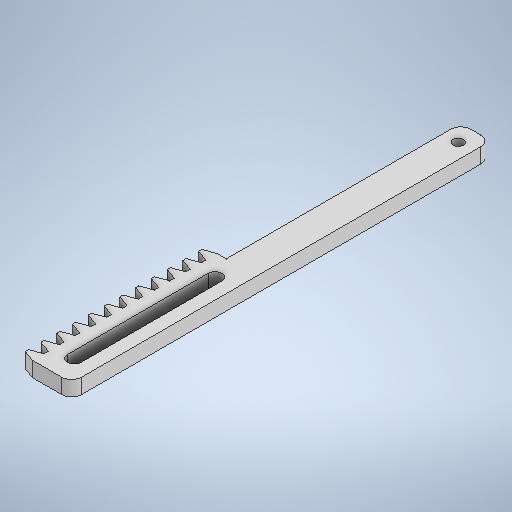
# Autodesk Inventor part: cremallera_v2
Saved by Autodesk Inventor 2025.2 (Build 292293000, 293)
## iProperties
Created: 2025-04-03
Part Number: cremallera_v2
Material: Generic
Document SubType Name: Modeling
Designer: cdavi
Density: 1 g/cm^3
Appearance: Default
Author: cdavi
Autodesk Inventor part; units mm, degrees
ref_plane "YZ Plane" through (0, 0, 0) normal (1, 0, 0) x (0, 1, 0)
ref_plane "XZ Plane" through (0, 0, 0) normal (0, 1, 0) x (-1, 0, 0)
ref_plane "XY Plane" through (0, 0, 0) normal (0, 0, 1) x (1, 0, 0)
sketch "Sketch1" plane through (0, 0, 0) normal (0, 1, 0) x (-1, 0, 0)
  line L0 (4.808, 48.5926) -> (7.058, 47.7737)
  line L1 (4.808, 49.4815) -> (4.808, 48.5926)
  line L2 (4.808, 49.4815) -> (7.058, 50.2996)
  line L3 (7.058, 50.2996) -> (7.058, 50.9144)
  line L4 (4.808, 51.7333) -> (7.058, 50.9144)
  line L5 (4.808, 52.6222) -> (4.808, 51.7333)
  line L6 (4.808, 52.6222) -> (7.058, 53.4403)
  line L7 (7.058, 53.4403) -> (7.058, 54.0552)
  line L8 (4.808, 54.8741) -> (7.058, 54.0552)
  line L9 (4.808, 55.763) -> (4.808, 54.8741)
  line L10 (4.808, 55.763) -> (7.058, 56.581)
  line L11 (7.058, 56.581) -> (7.058, 57.1959)
  line L12 (4.808, 58.0148) -> (7.058, 57.1959)
  line L13 (4.808, 58.9037) -> (4.808, 58.0148)
  line L14 (4.808, 58.9037) -> (7.058, 59.7218)
  line L15 (7.058, 59.7218) -> (7.058, 60.3366)
  line L16 (4.808, 61.1556) -> (7.058, 60.3366)
  line L17 (4.808, 62.0444) -> (4.808, 61.1556)
  line L18 (4.808, 62.0444) -> (7.058, 62.8625)
  line L19 (7.058, 62.8625) -> (7.058, 63.4774)
  line L20 (4.808, 64.2963) -> (7.058, 63.4774)
  line L21 (4.808, 65.1852) -> (4.808, 64.2963)
  line L22 (4.808, 65.1852) -> (7.058, 66.0033)
  line L23 (7.058, 66.0033) -> (7.058, 66.6181)
  line L24 (4.808, 67.437) -> (7.058, 66.6181)
  line L25 (4.808, 68.3259) -> (4.808, 67.437)
  line L26 (4.808, 68.3259) -> (7.058, 69.144)
  line L27 (7.058, 69.144) -> (7.058, 69.7588)
  line L28 (4.808, 70.5778) -> (7.058, 69.7588)
  line L29 (4.808, 71.4667) -> (4.808, 70.5778)
  line L30 (4.808, 71.4667) -> (7.058, 72.2847)
  line L31 (7.058, 72.2847) -> (7.058, 72.8996)
  line L32 (4.808, 73.7185) -> (7.058, 72.8996)
  line L33 (4.808, 74.6074) -> (4.808, 73.7185)
  line L34 (4.808, 74.6074) -> (7.058, 75.4255)
  line L35 (7.058, 75.4255) -> (7.058, 76.0403)
  line L36 (4.808, 76.8593) -> (7.058, 76.0403)
  line L37 (4.808, 77.7481) -> (4.808, 76.8593)
  line L38 (4.808, 77.7481) -> (7.058, 78.5662)
  line L39 (7.058, 78.5662) -> (7.058, 79.1811)
  line L40 (4.808, 80) -> (7.058, 79.1811)
  line L41 (-3, 80) -> (4.808, 80)
  line L42 (-3, 80) -> (-3, -1.5)
  arc A0 (-3, -1.5) -> (-1, -3.5) centre (-1, -1.5) ccw
  line L43 (1, -3.5) -> (-1, -3.5)
  arc A1 (1, -3.5) -> (3, -1.5) centre (1, -1.5) ccw
  line L44 (3, 43.2) -> (3, -1.5)
  line L45 (4.808, 43.2) -> (7.058, 44.0181)
  line L46 (7.058, 44.0181) -> (7.058, 44.6329)
  line L47 (4.808, 45.4519) -> (7.058, 44.6329)
  line L48 (4.808, 46.3407) -> (4.808, 45.4519)
  line L49 (4.808, 46.3407) -> (7.058, 47.1588)
  line L50 (7.058, 47.1588) -> (7.058, 47.7737)
  circle A2 centre (0, 0) radius 1
  arc A3 (-0.392, 47.5) -> (2.308, 47.5) centre (0.958, 47.5) ccw
  line L51 (-0.392, 75.5) -> (-0.392, 47.5)
  arc A4 (2.308, 75.5) -> (-0.392, 75.5) centre (0.958, 75.5) ccw
  line L52 (2.308, 75.5) -> (2.308, 47.5)
  line L53 (3, 43.2) -> (4.808, 43.2)
  point P0 (4.808, 77.3037)
  point P1 (4.808, 49.037)
  point P2 (0.904, 80)
  dimension "d0" = 2.25
  dimension "d3" = 28
  dimension "d4" = 2.7
  dimension "d7" = 2.5
  dimension "d8" = 4.3
  dimension "d11" = 6
  dimension "d12" = 3
  dimension "d13" = 3.5
  dimension "d15" = 0.6149
  dimension "d16" = 0.8889
  dimension "d17" = 20
  dimension "d28" = 4.808
  dimension "d29" = 36.8
  dimension "d30" = 4.5
  dimension "d31" = 83.5
  dimension "d32" = 2
  dimension "d33" = 2
  dimension "d34" = 2
  dimension "d37" = 2.608
  dimension "d38" = 2
  constraints: 109 end point, 42 collinear, 27 parallel, 22 vertical, 8 point on circle, 7 tangent, 5 centre point, 3 midpoint, 2 vertical alignment, 1 coincident, 1 horizontal
  measures "d0" distance from line of L40.start L39
  measures "d3" distance of L51.start L51.end
  measures "d4" distance between parallel lines of L51 L52
  measures "d7" distance from line of L45.start L52
  measures "d8" vertical distance of L44.start A3.centre
  measures "d11" distance between parallel lines of L42 L44
  measures "d12" distance from line of L44 A2.centre
  measures "d13" distance from line of L43 A2.centre
  measures "d15" distance of L38.end L39.end
  measures "d16" distance of L37.start L36.start
  measures "d17" angle of L41 L40
  measures "d28" horizontal distance of point (0, 0) L45.start
  measures "d29" distance from line of L41 L45.start
  measures "d30" vertical distance of point (0.904, 80) A4.centre
  measures "d31" distance between parallel lines of L41 L43
  measures "d32" radius of A1
  measures "d33" radius of A0
  measures "d34" distance from line of L44 A1.centre
  measures "d37" distance between parallel lines of L42 L51
  measures "d38" diameter of A2
extrude "Extrusion1" add sketch "Sketch1" along normal blind 3
fillet "Fillet1" radius 2 1 edges at (3, 1.5, 80)
equation "\"d28\" = dist_finEngrane_tornilloSujetadorPilot"
equation "\"dist_finEngrane_tornilloSujetadorPilot\" = 4.808"
body "Solid1"
